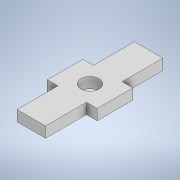
# Autodesk Inventor part: SoporteFotos
Saved by Autodesk Inventor 2020.2 (Build 242310000, 310)
## iProperties
Created: 2020-03-19
Part Number: SoporteFotos
Material: Generic
Document SubType Name: Modeling
Designer: ARQ SEVILLA R
Density: 1 g/cm^3
Appearance: Default
Author: ARQ SEVILLA R
Autodesk Inventor part; units mm, degrees
ref_plane "YZ Plane" through (0, 0, 0) normal (1, 0, 0) x (0, 1, 0)
ref_plane "XZ Plane" through (0, 0, 0) normal (0, 1, 0) x (-1, 0, 0)
ref_plane "XY Plane" through (0, 0, 0) normal (0, 0, 1) x (1, 0, 0)
sketch "Sketch1" plane through (0, 0, 0) normal (0, 1, 0) x (-1, 0, 0)
  line L0 (0, 0) -> (8, 0)
  line L1 (8, -31) -> (0, -31)
  circle A0 centre (4, -15.5) radius 2.55
  line L2 (8, 0) -> (8, -10.5)
  line L3 (8, -10.5) -> (11, -10.5)
  line L4 (11, -10.5) -> (11, -20.5)
  line L5 (11, -20.5) -> (8, -20.5)
  line L6 (8, 0) -> (8, -10.5)
  line L7 (8, -20.5) -> (8, -31)
  line L8 (4, 0) -> (4, -15.5) construction
  line L9 (0, -10.5) -> (-3, -10.5)
  line L10 (-3, -10.5) -> (-3, -20.5)
  line L11 (-3, -20.5) -> (0, -20.5)
  line L12 (0, -31) -> (0, -20.5)
  line L13 (0, -10.5) -> (0, 0)
  dimension "d0" = 8
  dimension "d1" = 31
  dimension "d2" = 5.1
  dimension "d3" = 10.5
  dimension "d4" = 3
  dimension "d5" = 10
  constraints: 28 end point, 6 perpendicular, 5 parallel, 4 symmetric about line, 1 centre point, 1 horizontal, 1 midpoint, 1 vertical
  measures "d0" distance of L1.start L1.end
  measures "d1" distance of L0.end L1.start
  measures "d2" diameter of A0
  measures "d3" distance of L0.end L2.end
  measures "d4" distance of L2.end L3.end
  measures "d5" distance of L3.end L4.end
extrude "Extrusion1" add sketch "Sketch1" along normal blind 3
sketch "Sketch2" plane through (0, 3, 0) normal (0, 1, 0) x (1, 0, 0)
  line L0 (0, 0) -> (0, 10.5) projected
  line L1 (0, 0) -> (0, -1)
  line L2 (0, -1) -> (-8, -1)
  line L3 (-8, 0) -> (0, 0) projected
  line L4 (-8, -1) -> (-8, 0)
  line L5 (0, 20.5) -> (0, 31) projected
  line L6 (0, 31) -> (0, 32)
  line L7 (0, 32) -> (-8, 32)
  line L8 (-8, 32) -> (-8, 31)
  line L9 (-8, 31) -> (-8, 20.5) projected
  line L10 (0, 31) -> (-8, 31) projected
  line L11 (-8, 31) -> (0, 31)
  dimension "d8" = 1
  dimension "d9" = 1
  constraints: 14 end point, 4 perpendicular, 2 vertical, 1 collinear
  measures "d8" distance of L0.start L1.end
  measures "d9" distance of L5.end L6.end
extrude "Extrusion2" add sketch "Sketch2" against normal up to surface (3 mm away)
body "Solid1"
